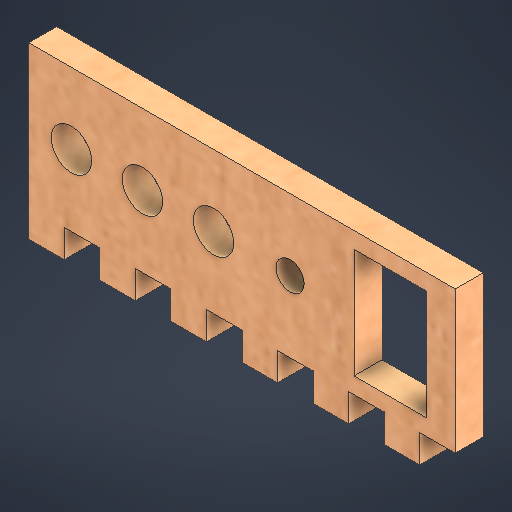
# Autodesk Inventor part: control_panel
Saved by Autodesk Inventor 2026 (Build 300175050, 175E)
## iProperties
Created: 2025-06-09
Part Number: control_panel
Material: Generic
Document SubType Name: Modeling
Designer: satom
Density: 1 g/cm^3
Appearance: Default
Author: satom
Autodesk Inventor part; units mm, degrees
ref_plane "YZ Plane" through (0, 0, 0) normal (1, 0, 0) x (0, 1, 0)
ref_plane "XZ Plane" through (0, 0, 0) normal (0, 1, 0) x (-1, 0, 0)
ref_plane "XY Plane" through (0, 0, 0) normal (0, 0, 1) x (1, 0, 0)
sketch "Sketch1" plane through (0, 0, 0) normal (0, 0, 1) x (1, 0, 0)
  line L0 (0, 0) -> (6.35, 0)
  line L1 (6.35, 0) -> (6.35, 5)
  line L2 (0, 5) -> (0, 0)
  line L3 (12.7, 0) -> (19.05, 0)
  line L4 (19.05, 0) -> (19.05, 5)
  line L5 (12.7, 5) -> (12.7, 0)
  line L6 (25.4, 0) -> (31.75, 0)
  line L7 (31.75, 0) -> (31.75, 5)
  line L8 (25.4, 5) -> (25.4, 0)
  line L9 (38.1, 0) -> (44.45, 0)
  line L10 (44.45, 0) -> (44.45, 5)
  line L11 (38.1, 5) -> (38.1, 0)
  line L12 (50.8, 0) -> (57.15, 0)
  line L13 (57.15, 0) -> (57.15, 5)
  line L14 (50.8, 5) -> (50.8, 0)
  line L15 (63.5, 0) -> (69.85, 0)
  line L16 (69.85, 0) -> (69.85, 5)
  line L17 (63.5, 5) -> (63.5, 0)
  line L18 (76.2, 5) -> (76.2, 30.4)
  line L19 (76.2, 30.4) -> (0, 30.4)
  line L20 (0, 30.4) -> (0, 5)
  line L21 (6.35, 5) -> (12.7, 5)
  line L22 (19.05, 5) -> (25.4, 5)
  line L23 (31.75, 5) -> (38.1, 5)
  line L24 (44.45, 5) -> (50.8, 5)
  line L25 (57.15, 5) -> (63.5, 5)
  line L26 (69.85, 5) -> (76.2, 5)
  dimension "d3" = 6.35
  dimension "d4" = 5
  dimension "d7" = 12.7
  dimension "d12" = 76.2
  dimension "d13" = 25.4
  constraints: 54 end point, 8 horizontal, 8 parallel, 7 perpendicular, 1 collinear, 34 other
  measures "d3" distance of L0.start L0.end
  measures "d4" distance of L2.start L0.start
  measures "d7" distance of L1.end L4.end
  measures "d12" distance of L18.end L19.end
  measures "d13" distance of L19.end L2.start
extrude "Extrusion1" add sketch "Sketch1" along normal blind 5
sketch "Sketch2" plane through (0, 0, 5) normal (0, 0, 1) x (1, 0, 0)
  line L0 (71.12, 27.5) -> (58.12, 27.5)
  line L1 (58.12, 27.5) -> (58.12, 7.9)
  line L2 (58.12, 7.9) -> (71.12, 7.9)
  line L3 (71.12, 7.9) -> (71.12, 27.5)
  line L4 (76.2, 17.7) -> (0.6797, 17.7)
  line L5 (76.2, 5) -> (76.2, 30.4) projected
  point P0 (0, 0)
  point P1 (71.12, 17.7)
  dimension "d16" = 13
  dimension "d17" = 19.6
  dimension "d20" = 5.08
  constraints: 10 end point, 3 horizontal, 2 parallel, 1 midpoint, 1 perpendicular, 1 point on line
  measures "d16" distance of L1.end L2.end
  measures "d17" distance of L2.end L0.start
  measures "d20" distance between parallel lines of L5 L3
extrude "Switch" cut sketch "Sketch2" against normal blind 5
sketch "Sketch3" plane through (0, 0, 5) normal (0, 0, 1) x (1, 0, 0)
  circle A0 centre (46.69, 17.7) radius 2.5
  line L0 (76.2, 5) -> (76.2, 30.4) construction
  line L1 (58.12, 7.9) -> (58.12, 27.5) construction
  line L2 (76.2, 17.7) -> (0, 17.7) construction
  line L3 (0, 30.4) -> (0, 0) construction
  dimension "d23" = 5
  dimension "d24" = 11.43
  constraints: 2 end point, 2 horizontal, 2 point on line, 1 centre point, 1 midpoint
  measures "d23" diameter of A0
  measures "d24" distance from line of L1 A0.centre
extrude "LED" cut sketch "Sketch3" against normal blind 5
sketch "Sketch4" plane through (0, 0, 5) normal (0, 0, 1) x (1, 0, 0)
  circle A0 centre (33.02, 17.7) radius 3.6
  line L0 (76.2, 5) -> (76.2, 30.4) construction
  line L1 (76.2, 17.7) -> (0, 17.7) construction
  circle A1 centre (20.32, 17.7) radius 3.6
  circle A2 centre (7.62, 17.7) radius 3.6
  line L2 (0, 30.4) -> (0, 0) projected
  dimension "d27" = 7.2
  dimension "d28" = 7.2
  dimension "d29" = 7.2
  dimension "d30" = 12.7
  dimension "d31" = 12.7
  dimension "d33" = 7.62
  constraints: 3 centre point, 3 point on line, 2 end point, 1 horizontal, 1 midpoint
  measures "d27" diameter of A0
  measures "d28" diameter of A1
  measures "d29" diameter of A2
  measures "d30" distance of A2.centre A1.centre
  measures "d31" distance of A0.centre A1.centre
  measures "d33" distance from line of L2 A2.centre
extrude "Buttons" cut sketch "Sketch4" against normal blind 5
equation "\"d4\" = hardboard_thickness"
equation "\"d14\" = hardboard_thickness"
equation "\"d21\" = hardboard_thickness"
equation "\"d25\" = hardboard_thickness"
equation "\"d34\" = hardboard_thickness"
equation "\"m3_heat_set_insert\" = 4"
equation "\"m3_clearance\" = 3.4"
equation "\"m3_heat_set_depth\" = 7"
equation "\"robot_diameter\" = 354"
equation "\"hardboard_thickness\" = 5"
body "Solid1"
